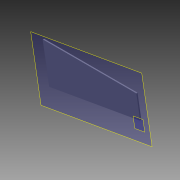
# Autodesk Inventor part: Panel_side
Saved by Autodesk Inventor 2013 (Build 170138000, 138)
## iProperties
Created: 2013-02-01
Part Number: Panel_side
Material: Aluminum 6061
Document SubType Name: Modeling
Designer: xylzlyx
Density: 1 g/cm^3
Author: xylzlyx
Autodesk Inventor part; units mm, degrees
ref_plane "YZ Plane" through (0, 0, 0) normal (1, 0, 0) x (0, 1, 0)
ref_plane "XZ Plane" through (0, 0, 0) normal (0, 1, 0) x (-1, 0, 0)
ref_plane "XY Plane" through (0, 0, 0) normal (0, 0, 1) x (1, 0, 0)
ref_plane "Work Plane2" through (0, 0, -10) normal (0, 0, -1) x (-0.9848078, -0.1736482, 0)
ref_plane "Work Plane1" through (0, 0, 0) normal (0, 0, -1) x (-0.9848078, -0.1736482, 0)
sketch "Sketch1" plane through (0, 0, -10) normal (0, 0, -1) x (-0.9848078, -0.1736482, 0)
  line L0 (4, 54.6856) -> (7, 54.6856) construction
  line L1 (7, 54.6856) -> (7, 0) construction
  line L2 (7, 0) -> (4, 0) construction
  line L3 (4, 0) -> (4, 54.6856) construction
  line L4 (246.7229, -3) -> (0, -3) construction
  line L5 (0, -3) -> (0, 0) construction
  line L6 (0, 0) -> (246.7229, 0) construction
  line L7 (246.7229, 0) -> (246.7229, -3) construction
  line L8 (0, 57.5265) -> (246.2019, 100.9386) construction
  line L9 (246.2019, 100.9386) -> (246.7229, 97.9842) construction
  line L10 (246.7229, 97.9842) -> (0.5209, 54.5721) construction
  line L11 (0.5209, 54.5721) -> (0, 57.5265) construction
  line L12 (242.7229, 94.2788) -> (242.7229, 0) construction
  line L13 (242.7229, 0) -> (239.7229, 0) construction
  line L14 (239.7229, 0) -> (239.7229, 94.2788) construction
  line L15 (239.7229, 94.2788) -> (242.7229, 94.2788) construction
  line L16 (239.7229, 96.7499) -> (239.7229, 0)
  line L17 (239.7229, 0) -> (7, 0)
  line L18 (7, 55.7145) -> (7, 0)
  line L19 (7, 55.7145) -> (239.7229, 96.7499)
  constraints: 40 end point, 6 horizontal, 6 vertical, 3 collinear, 2 coincident, 2 point on line, 2 vertical alignment, 1 parallel, 19 other
extrude "Extrusion1" add sketch "Sketch1" along normal blind 3
fillet "Corners" radius 1 4 edges at (-252.8814, 53.6526, -11.5) (-236.081, -41.6274, -11.5) (-6.8937, -1.2155, -11.5) (-16.5684, 53.6526, -11.5)
body "Solid1"
